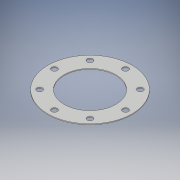
# Autodesk Inventor part: Upper Cylinder Packing
Saved by Autodesk Inventor 2017 (Build 210142000, 142)
## iProperties
Created: 2018-10-30
Part Number: Upper Cylinder Packing
Material: Generic
Document SubType Name: Modeling
Designer: 623516
Density: 1 g/cm^3
Appearance: Default
Author: 623516
Autodesk Inventor part; units mm, degrees
ref_plane "YZ Plane" through (0, 0, 0) normal (1, 0, 0) x (0, 1, 0)
ref_plane "XZ Plane" through (0, 0, 0) normal (0, 1, 0) x (-1, 0, 0)
ref_plane "XY Plane" through (0, 0, 0) normal (0, 0, 1) x (1, 0, 0)
sketch "Sketch1" plane through (0, 0, 0) normal (0, 1, 0) x (-1, 0, 0)
  circle A0 centre (0, 0) radius 26
  circle A1 centre (0, 0) radius 16
  circle A2 centre (0, 0) radius 22 construction
  circle A3 centre (22, 0) radius 1.75 construction
  circle A4 centre (0, -22) radius 1.75 construction
  circle A5 centre (-22, 0) radius 1.75 construction
  circle A6 centre (-22, 0) radius 1.75
  circle A7 centre (0, -22) radius 1.75
  circle A8 centre (22, 0) radius 1.75
  line L0 (0, 22) -> (0, 0) construction
  line L1 (0, 0) -> (39.0381, 0) construction
  line L2 (0, 0) -> (31.228, -31.228) construction
  line L3 (0, 0) -> (44.1631, 0) construction
  circle A9 centre (15.5563, -15.5563) radius 1.75
  line L4 (0, 0) -> (-25.3717, -25.3717) construction
  line L5 (0, 0) -> (-36.3161, 0) construction
  circle A10 centre (-15.5563, -15.5563) radius 1.75
  circle A11 centre (0, 22) radius 1.75
  line L6 (0, 0) -> (18.3848, 18.3848) construction
  line L7 (0, 0) -> (26, 0) construction
  line L8 (0, 0) -> (-18.3848, 18.3848) construction
  line L9 (0, 0) -> (26, 0) construction
  circle A12 centre (15.5563, 15.5563) radius 1.75
  circle A13 centre (-15.5563, 15.5563) radius 1.75
  dimension "d2" = 44
  dimension "d1" = 32
  dimension "d3" = 3.5
  dimension "d4" = 3.5
  dimension "d5" = 3.5
  dimension "d34" = 45
  dimension "d35" = 3.5
  dimension "d36" = 45
  dimension "d37" = 3.5
  dimension "d38" = 52
  dimension "d39" = 31.228
  dimension "d40" = 27.6041
  dimension "d41" = 0
  dimension "d42" = 22
  dimension "d43" = 22
  dimension "d44" = 0
  dimension "d45" = 25.3717
  dimension "d46" = 25.6793
  dimension "d49" = 3.5
  dimension "d51" = 45
  dimension "d52" = 135
  dimension "d53" = 3.5
  dimension "d54" = 3.5
  constraints: 20 end point, 13 centre point, 7 coincident, 5 horizontal, 4 point on line, 3 concentric, 3 equal length, 2 point on circle, 1 vertical, 9 other
  measures "d1" diameter of A1
  measures "d3" diameter of A3
  measures "d4" diameter of A4
  measures "d5" diameter of A5
  measures "d34" angle of L2 L3
  measures "d35" diameter of A9
  measures "d36" angle of L5 L4
  measures "d37" diameter of A10
  measures "d38" diameter of A0
  measures "d39" distance from line of L3.end L2
  measures "d40" distance from line of L1.end L2
  measures "d41" distance from line of A8.centre L1
  measures "d42" distance from line of L0.start L3
  measures "d43" distance from line of A4.centre L3
  measures "d44" distance from line of A5.centre L3
  measures "d45" distance from line of L4.end L3
  measures "d46" distance from line of L5.end L2
  measures "d49" diameter of A11
  measures "d51" angle of L7 L6
  measures "d52" angle of L9 L8
  measures "d53" diameter of A12
  measures "d54" diameter of A13
extrude "Extrusion5" add sketch "Sketch1" along normal blind 0.5
body "Solid4"
